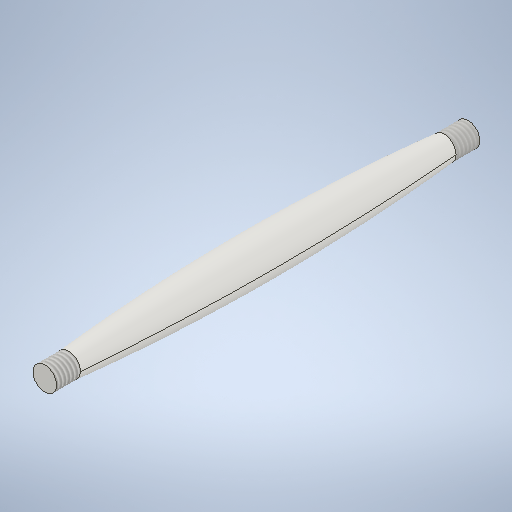
# Autodesk Inventor part: 16A - Con Rod
Saved by Autodesk Inventor 2025.2 (Build 292293000, 293)
## iProperties
Created: 2025-06-12
Part Number: 16A - Con Rod
Material: Steel AISI 1020 107 HR
Document SubType Name: Modeling
Designer: bless
Density: 7.87 g/cm^3
Appearance: Steel
Author: bless
Autodesk Inventor part; units mm, degrees
ref_plane "YZ Plane" through (0, 0, 0) normal (1, 0, 0) x (0, 1, 0)
sketch "Sketch1" plane through (0, 0, 0) normal (0, 0, 1) x (1, 0, 0)
  circle A0 centre (0, 0) radius 5
  dimension "d0" = 10
  constraints: 1 centre point, 1 coincident
  measures "d0" diameter of A0
ref_plane "Work Plane1" through (0, 0, 47.25) normal (0, 0, 1) x (1, 0, 0)
ref_plane "Work Plane2" through (0, 0, -47.25) normal (0, 0, 1) x (1, 0, 0)
sketch "Sketch2" plane through (0, 0, -47.25) normal (0, 0, 1) x (1, 0, 0)
  circle A0 centre (0, 0) radius 3
  dimension "d3" = 6
  constraints: 1 centre point, 1 coincident
  measures "d3" diameter of A0
sketch "Sketch3" plane through (0, 0, 47.25) normal (0, 0, 1) x (1, 0, 0)
  circle A0 centre (0, 0) radius 3
  dimension "d4" = 6
  constraints: 1 centre point, 1 coincident
  measures "d4" diameter of A0
loft "Loft1" add profiles "Sketch3", "Sketch1", "Sketch2"
sketch "Sketch4" plane through (0, 0, 47.25) normal (0, 0, 1) x (1, 0, 0)
  circle A0 centre (0, 0) radius 3 projected
  point P0 (3, 0)
  constraints: 1 horizontal alignment
extrude "Extrusion1" add sketch "Sketch4" along normal blind 6
sketch "Sketch5" plane through (0, 0, -47.25) normal (0, 0, -1) x (-1, 0, 0)
  circle A0 centre (0, 0) radius 3 projected
  point P0 (-3, 0)
  constraints: 1 horizontal alignment
extrude "Extrusion2" add sketch "Sketch5" along normal blind 6
thread "Thread1" size "M6x1" class "6g" standard "ANSI Metric M Profile" length 6
thread "Thread2" size "M6x1" class "6g" standard "ANSI Metric M Profile" length 6
body "Solid1"
